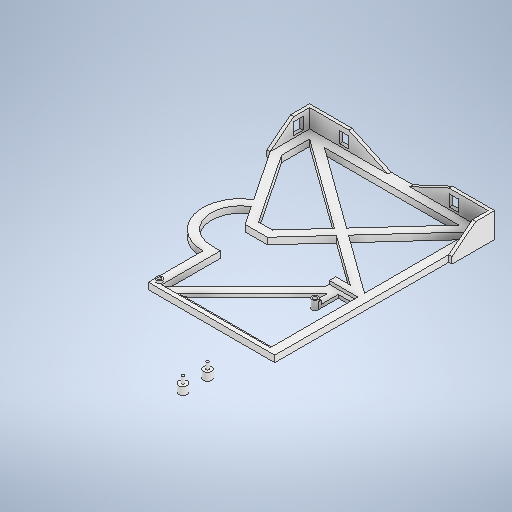
# Autodesk Inventor part: OscarNoring240sSkalV.1Städad
Saved by Autodesk Inventor 2025.2 (Build 292293000, 293)
## iProperties
Created: 2024-12-07
Part Number: OscarNoring240sSkalV.1Städad
Material: PBT Plastic
Document SubType Name: Modeling
Designer: oscar_j04e9wl
Density: 1.31 g/cm^3
Appearance: Smooth - White
Author: oscar_j04e9wl
Autodesk Inventor part; units mm, degrees
ref_plane "YZ Plane" through (0, 0, 0) normal (1, 0, 0) x (0, 1, 0)
ref_plane "XZ Plane" through (0, 0, 0) normal (0, 1, 0) x (-1, 0, 0)
ref_plane "XY Plane" through (0, 0, 0) normal (0, 0, 1) x (1, 0, 0)
sketch "Sketch1" plane through (0, 0, 0) normal (0, 1, 0) x (-1, 0, 0)
  line L0 (0, 0) -> (0, -52.786)
  line L1 (0, -52.786) -> (82, -52.786)
  line L2 (82, -52.786) -> (82, -34.682)
  line L3 (0, 0) -> (0, 5)
  line L4 (0, 5) -> (0, 45.214)
  line L5 (0, 45.214) -> (58, 45.214)
  line L6 (58, 45.214) -> (58, 20.214)
  line L7 (82, -34.682) -> (58.8095, -0.0012)
  line L8 (58.8095, -0.0012) -> (48.5795, -0.0012)
  line L9 (54, 16.214) -> (54, 41.214)
  line L10 (54, 41.214) -> (4, 41.214)
  line L11 (4, 41.214) -> (4, 4.9997)
  line L12 (4, 4.9997) -> (4, -0.0003)
  line L13 (4, -0.0003) -> (4, -48.786)
  line L14 (4, -48.786) -> (78, -48.786)
  line L15 (78, -48.786) -> (78, -35.8961)
  line L16 (78, -35.8961) -> (56.6724, -4.0012)
  line L17 (56.6724, -4.0012) -> (50.3428, -4.0012)
  arc A0 (66.676, -11.7654) -> (58, 20.214) centre (58.0504, 3.0611) ccw
  line L18 (54, 16.214) -> (58.0272, 16.214)
  arc A1 (64.4526, -8.4403) -> (58.0272, 16.214) centre (58.0714, 3.0611) ccw
  line L19 (48.5795, -0.0012) -> (4, -48.786)
  line L20 (50.3428, -4.0012) -> (9.4185, -48.786)
  line L21 (4, -0.0003) -> (71.192, -48.786)
  line L22 (4, -0.0003) -> (17.14, -0.0003)
  line L23 (4, 4.9997) -> (17.14, 4.9997)
  line L24 (17.14, -0.0003) -> (17.14, 4.9997)
  line L25 (54, 41.214) -> (17.14, 4.9997)
  line L26 (48.2925, 41.214) -> (11.4325, 4.9997)
  line L27 (13.95, 4.9997) -> (13.95, 14.2137)
  line L28 (13.95, 14.2137) -> (11.05, 14.2137)
  line L29 (11.05, 14.2137) -> (11.05, 4.9997)
  circle A2 centre (12.5, 14.2137) radius 1.45
  circle A3 centre (12.5, 14.2137) radius 0.9
  line L30 (78, -48.786) -> (10.57, -0.0003)
  circle A4 centre (56, 42.214) radius 1.45
  circle A5 centre (56, 42.214) radius 0.9
  circle A6 centre (9.4185, 66.6658) radius 2
  line L31 (5.6424, 72.3128) -> (12.2144, 72.3128) construction
  circle A7 centre (9.4185, 77.9599) radius 2
  point P0 (34.0568, -21.8235)
  point P1 (30.7995, -19.4584)
  point P2 (36.7141, -18.9156)
  point P3 (33.4521, -16.5555)
  point P4 (13.95, 7.4731)
  dimension "d0" = 52.786
  dimension "d1" = 82
  dimension "d2" = 18.104
  dimension "d3" = 5
  dimension "d4" = 40.214
  dimension "d5" = 58
  dimension "d6" = 25
  dimension "d7" = 146.23
  dimension "d8" = 41.72
  dimension "d9" = 10.23
  dimension "d12" = 4
  dimension "d13" = 17.153
  dimension "d14" = 27.568
  dimension "d15" = 25
  dimension "d16" = 13.153
  dimension "d17" = 4
  dimension "d18" = 0
  dimension "d19" = 4
  dimension "d20" = 6.808
  dimension "d21" = 83.035
  dimension "d22" = 13.14
  dimension "d23" = 5
  dimension "d24" = 4
  dimension "d25" = 9.214
  dimension "d26" = 3.19
  dimension "d27" = 2.9
  dimension "d28" = 1.8
  dimension "d29" = 3
  dimension "d30" = 2
  dimension "d31" = 2.9
  dimension "d32" = 1.8
  dimension "d33" = 4
  constraints: 64 end point, 8 point on line, 7 centre point, 7 horizontal, 6 perpendicular, 5 vertical, 4 point on circle, 2 coincident, 2 midpoint, 2 parallel, 1 symmetric about line, 12 other
  measures "d0" distance of L0.start L0.end
  measures "d1" distance of L0.end L1.end
  measures "d2" distance of L1.end L2.end
  measures "d3" distance of L0.start L3.end
  measures "d4" distance of L3.end L4.end
  measures "d5" distance of L4.end L5.end
  measures "d6" distance of L5.end L6.end
  measures "d7" angle of L2 L7
  measures "d8" distance of L2.end L7.end
  measures "d9" distance of L7.end L8.end
  measures "d12" distance between parallel lines of L5 L10
  measures "d13" radius of A0
  measures "d14" distance of L2.end A0.start
  measures "d15" distance of L9.start L9.end
  measures "d16" radius of A1
  measures "d17" distance of A0.start A1.start
  measures "d18" vertical distance of A0.centre A1.centre
  measures "d19" distance between parallel lines of L19 L20
  measures "d20" distance of L14.end L21.end
  measures "d21" distance of L12.end L21.end
  measures "d22" distance of L12.end L22.end
  measures "d23" distance between parallel lines of L22 L23
  measures "d24" distance between parallel lines of L25 L26
  measures "d25" distance of L27.start L27.end
  measures "d26" distance of L23.end L27.start
  measures "d27" distance of L27.end L28.end
  measures "d28" diameter of A3
  measures "d29" distance from line of L5 A4.centre
  measures "d30" distance from line of L6 A4.centre
  measures "d31" diameter of A4
  measures "d32" diameter of A5
  measures "d33" diameter of A6
extrude "Extrusion1" add sketch "Sketch1" along normal blind 3 contours L3 L4 L5 L6 A0 L7 L2 L1 L0 | L30 L20 L21 L19 | L19 L21 L22 L30 | L25 L23 L27 L26 L10 | L21 L20 L14 L19 | L30 L14 L21 L20 | L22 L12 L23 L24 | L27 L23 L26 | L26 L23 L29 A2 L27
extrude "Extrusion2" add sketch "Sketch1" along normal blind 4 contours A2 L28 A3 | L28 A3 A2 | A4
sketch "Sketch4" plane through (0, 3, 0) normal (0, 1, 0) x (1, 0, 0)
  line L0 (-4, -4.9997) -> (-4, -41.214) projected
  line L1 (-4, -41.214) -> (-54, -41.214)
  line L2 (-54, -41.214) -> (-54, -43.214)
  line L3 (-54, -43.214) -> (-4, -43.214)
  line L4 (-4, -43.214) -> (-4, -41.214)
  line L5 (-54, -41.214) -> (-54, -16.214) projected
  line L6 (-17.14, -4.9997) -> (-17.14, -2.9997)
  line L7 (-17.14, 0.0003) -> (-17.14, -4.9997) projected
  line L8 (-17.14, -2.9997) -> (-4, -2.9997)
  line L9 (-4, -2.9997) -> (-4, -4.9997)
  line L10 (-11.05, -14.2137) -> (-11.05, -4.9997) projected
  line L11 (-4, -4.9997) -> (-11.05, -4.9997)
  line L12 (-11.05, -4.9997) -> (-11.05, -12.7497)
  line L13 (-11.05, -14.2137) -> (-11.05, -4.9997) projected
  line L14 (-11.05, -12.7497) -> (-13.95, -12.7497)
  line L15 (-13.95, -7.4731) -> (-13.95, -14.2137) projected
  line L16 (-13.95, -7.4731) -> (-13.95, -12.7497)
  line L17 (-48.2925, -41.214) -> (-13.95, -7.4731) projected
  line L18 (-13.95, -7.4731) -> (-48.2925, -41.214)
  line L19 (-17.14, -4.9997) -> (-54, -41.214) projected
  line L20 (-17.14, -4.9997) -> (-54, -41.214)
  point P0 (0, 0)
  dimension "d38" = 2
  dimension "d39" = 0
  dimension "d40" = 2
  dimension "d41" = 7.75
  constraints: 26 end point, 4 point on line, 3 collinear, 3 horizontal, 2 parallel, 2 perpendicular
  measures "d38" distance between parallel lines of L1 L3
  measures "d39" distance between parallel lines of L5 L2
  measures "d40" distance of L6.start L6.end
  measures "d41" distance of L10.end L12.end
extrude "Extrusion3" cut sketch "Sketch4" against normal blind 1.5 contours L11 L10 L14 L15 L17 L1 L19 L6 L8 L9 | L4 L3 L2 L1
sketch "Sketch5" plane through (0, 0, -52.786) normal (0, 0, -1) x (-1, 0, 0)
  line L0 (0, 0) -> (0, 3) projected
  line L1 (82, 0) -> (82, 3) projected
  line L2 (0, 0) -> (82, 0)
  line L3 (82, 0) -> (82, 3)
  line L4 (82, 3) -> (0, 3)
  line L5 (0, 3) -> (0, 0)
  line L6 (0, 3) -> (0, 11.5)
  line L7 (0, 11.5) -> (17.94, 11.5)
  line L8 (17.94, 11.5) -> (36.0439, 3)
  line L9 (17.94, 4) -> (13.74, 4)
  line L10 (13.74, 4) -> (13.74, 9.2)
  line L11 (13.74, 9.2) -> (17.94, 9.2)
  line L12 (17.94, 9.2) -> (17.94, 4)
  line L13 (41, 0) -> (41, 9.2) construction
  line L14 (82, 3) -> (82, 11.5)
  line L15 (82, 11.5) -> (64.06, 11.5)
  line L16 (64.06, 11.5) -> (45.9561, 3)
  line L17 (64.06, 4) -> (68.26, 4)
  line L18 (68.26, 4) -> (68.26, 9.2)
  line L19 (68.26, 9.2) -> (64.06, 9.2)
  line L20 (64.06, 9.2) -> (64.06, 4)
  point P0 (82, 0)
  point P1 (82, 3)
  point P2 (45.9561, 3)
  dimension "d44" = 8.5
  dimension "d45" = 17.94
  dimension "d46" = 20
  dimension "d47" = 2.3
  dimension "d48" = 2.3
  dimension "d49" = 5.2
  dimension "d50" = 4.2
  constraints: 38 end point, 9 symmetric about line, 4 parallel, 3 horizontal, 3 perpendicular, 1 midpoint, 1 point on line, 1 vertical
  measures "d44" distance of L4.end L6.end
  measures "d45" distance of L6.end L7.end
  measures "d46" distance of L7.end L8.end
  measures "d47" distance between parallel lines of L7 L11
  measures "d48" distance of L7.end L11.end
  measures "d49" distance between parallel lines of L11 L9
  measures "d50" distance between parallel lines of L10 L12
extrude "Extrusion4" add sketch "Sketch5" along normal blind 1.5
sketch "Sketch6" plane through (0, 0, 45.214) normal (1, 0, 0) x (0, 0, -1)
  line L0 (99.5, 0) -> (99.5, 11.5) projected
  line L1 (0, 3) -> (98, 3) projected
  line L2 (99.5, 0) -> (79.896, 0)
  line L3 (79.896, 0) -> (79.896, 3)
  line L4 (79.896, 3) -> (99.5, 3)
  line L5 (99.5, 3) -> (99.5, 0)
  line L6 (98, 11.5) -> (99.5, 11.5) projected
  line L7 (99.5, 11.5) -> (90.8005, 11.5)
  line L8 (79.896, 3) -> (90.8005, 11.5)
  point P0 (45.214, 0)
  dimension "d53" = 19.604
  dimension "d55" = 13.826
  constraints: 12 end point, 2 horizontal, 2 parallel, 1 perpendicular, 1 point on line
  measures "d53" distance between parallel lines of L3 L0
  measures "d55" distance of L3.end L7.end
extrude "Extrusion5" add sketch "Sketch6" along normal blind 1.5
sketch "Sketch7" plane through (-82, 0, -34.682) normal (-1, 0, 0) x (0, 0, 1)
  line L0 (-19.604, 0) -> (-19.604, 11.5) projected
  line L1 (79.896, 0) -> (0, 0) projected
  line L2 (-19.604, 0) -> (0, 0)
  line L3 (0, 0) -> (0, 3)
  line L4 (-18.104, 11.5) -> (-10.9045, 11.5) projected
  line L5 (0, 3) -> (-10.9045, 11.5)
  line L6 (-10.9045, 11.5) -> (-19.604, 11.5)
  line L7 (-19.604, 0) -> (-19.604, 11.5)
  line L8 (-10.604, 4) -> (-15.104, 4)
  line L9 (-15.104, 4) -> (-15.104, 9.5)
  line L10 (-15.104, 9.5) -> (-10.604, 9.5)
  line L11 (-10.604, 9.5) -> (-10.604, 4)
  point P0 (34.682, 0)
  dimension "d58" = 13.826
  dimension "d59" = 4.5
  dimension "d60" = 5.5
  dimension "d61" = 2
  dimension "d62" = 4.5
  constraints: 18 end point, 3 perpendicular, 2 horizontal, 2 parallel, 1 collinear
  measures "d58" distance of L3.end L4.end
  measures "d59" distance between parallel lines of L9 L11
  measures "d60" distance between parallel lines of L10 L8
  measures "d61" distance between parallel lines of L4 L10
  measures "d62" distance between parallel lines of L0 L9
extrude "Extrusion6" add sketch "Sketch7" along normal blind 1.5
extrude "Extrusion7" add sketch "Sketch1" along normal blind 3.5 contours A6 | A7
sketch "Sketch8" plane through (-9.4185, 3.5, 66.6658) normal (0, 1, 0) x (1, 0, 0)
  circle A0 centre (0, 0) radius 0.65
  line L0 (3.3606, -5.6379) -> (-2.349, -5.6379) construction
  circle A1 centre (0, 0) radius 2 construction
  circle A2 centre (0, -11.2758) radius 0.65
  point P0 (9.4185, 66.6658)
  dimension "d67" = 1.3
  dimension "d68" = 1.35
  constraints: 2 centre point, 2 end point, 1 horizontal, 1 symmetric about line, 1 other
  measures "d67" diameter of A0
  measures "d68" radial gap between concentric circles of A1 A0
extrude "Extrusion8" add sketch "Sketch8" along normal blind 3
equation "\"d31\" = d27"
equation "\"d32\" = d28"
body "Solid1"
